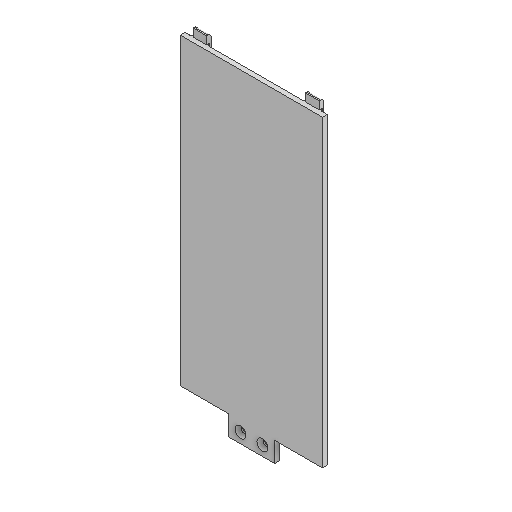
# Autodesk Inventor part: plate cover 2
Saved by Autodesk Inventor 2025.3 (Build 293356030, 356C)
## iProperties
Created: 2025-10-11
Part Number: plate cover 2
Material: 일반
Document SubType Name: Modeling
Designer: joseph
Density: 1 g/cm^3
Appearance: 기본값
Author: joseph
Autodesk Inventor part; units mm, degrees
ref_plane "YZ Plane" through (0, 0, 0) normal (1, 0, 0) x (0, 1, 0)
ref_plane "XZ Plane" through (0, 0, 0) normal (0, 1, 0) x (-1, 0, 0)
ref_plane "XY Plane" through (0, 0, 0) normal (0, 0, 1) x (1, 0, 0)
sketch "스케치1" plane through (0, 0, 0) normal (0, 0, 1) x (1, 0, 0)
  line L0 (0, 0) -> (90.5, 0)
  line L1 (90.5, 0) -> (90.5, 193.4)
  line L2 (90.5, 193.4) -> (0, 193.4)
  line L3 (0, 193.4) -> (0, 0)
  dimension "d0" = 90.5
  dimension "d1" = 193.4
  constraints: 8 end point, 2 parallel, 1 horizontal, 1 perpendicular
  measures "d0" distance of L2.end L1.end
  measures "d1" distance of L1.end L0.end
extrude "돌출1" add sketch "스케치1" along normal blind 3
sketch "스케치2" plane through (0, 0, 3) normal (0, 0, 1) x (1, 0, 0)
  line L0 (0, 0) -> (90.5, 0) projected
  line L1 (30.45, 0) -> (60.05, 0)
  line L2 (60.05, 0) -> (60.05, -12.8)
  line L3 (60.05, -12.8) -> (30.45, -12.8)
  line L4 (30.45, -12.8) -> (30.45, 0)
  circle A0 centre (38.25, -6.4) radius 1.5
  circle A1 centre (52.25, -6.4) radius 1.5
  point P0 (45.25, 0)
  dimension "d4" = 29.6
  dimension "d5" = 12.8
  dimension "d6" = 3
  dimension "d7" = 3
  dimension "d8" = 7.8
  dimension "d9" = 7.8
  constraints: 8 end point, 2 centre point, 2 midpoint, 2 parallel, 1 horizontal, 1 perpendicular, 1 point on line
  measures "d4" distance of L2.end L3.end
  measures "d5" distance of L1.end L2.end
  measures "d6" diameter of A0
  measures "d7" diameter of A1
  measures "d8" horizontal distance of L3.end A0.centre
  measures "d9" distance from line of L2 A1.centre
extrude "돌출2" add sketch "스케치2" against normal blind 3
sketch "스케치3" plane through (0, 193.4, 0) normal (0, 1, 0) x (1, 0, 0)
  line L0 (90.5, 0) -> (0, 0) projected
  line L1 (0, 0) -> (0, -3) projected
  line L2 (90.5, -3) -> (0, -3) projected
  line L3 (90.5, 0) -> (90.5, -3) projected
  line L4 (5.1, 0) -> (13.8, 0)
  line L5 (13.8, 0) -> (13.8, 2.8)
  line L6 (13.8, 2.8) -> (5.1, 2.8)
  line L7 (5.1, 2.8) -> (5.1, 0)
  line L8 (45.25, -3) -> (45.25, 0) construction
  line L9 (0, 0) -> (90.5, 0)
  line L10 (0, -3) -> (90.5, -3)
  line L11 (85.4, 0) -> (76.7, 0)
  line L12 (76.7, 0) -> (76.7, 2.8)
  line L13 (76.7, 2.8) -> (85.4, 2.8)
  line L14 (85.4, 2.8) -> (85.4, 0)
  dimension "d12" = 8.7
  dimension "d13" = 2.8
  dimension "d14" = 5.1
  constraints: 22 end point, 8 symmetric about line, 2 midpoint, 2 parallel, 2 point on line, 1 horizontal, 1 perpendicular
  measures "d12" distance of L6.end L5.end
  measures "d13" distance of L5.end L4.end
  measures "d14" horizontal distance of point (0, 0) L6.end
extrude "돌출3" add sketch "스케치3" against normal blind 20 contours L0 L12 L13 L14 | L0 L7 L6 L5
sketch "스케치4" plane through (0, 193.4, 3) normal (0, 1, 0) x (1, 0, 0)
  line L0 (5.1, 3) -> (5.1, 5.8) projected
  line L1 (13.8, 5.8) -> (13.8, 3) projected
  line L2 (5.1, 5.8) -> (13.8, 5.8)
  line L3 (13.8, 5.8) -> (13.8, 3)
  line L4 (13.8, 3) -> (5.1, 3)
  line L5 (5.1, 3) -> (5.1, 5.8)
  line L6 (85.4, 5.8) -> (76.7, 5.8) projected
  line L7 (76.7, 5.8) -> (85.4, 5.8)
  line L8 (85.4, 5.8) -> (85.4, 3)
  line L9 (85.4, 3) -> (76.7, 3)
  line L10 (76.7, 3) -> (76.7, 5.8)
  point P0 (0, 3)
  constraints: 16 end point, 4 parallel, 2 horizontal, 2 perpendicular, 1 point on line
extrude "돌출4" add sketch "스케치4" along normal blind 5
fillet "모깎기1" radius 2 8 edges at (9.45, 198.4, -2.8) (81.05, 198.4, -2.8) (5.1, 183.4, 0) (9.45, 173.4, 0) (13.8, 183.4, 0) (85.4, 183.4, 0) (81.05, 173.4, 0) (76.7, 183.4, 0)
fillet "모깎기2" radius 2 2 edges at (36.75, -6.4, 3) (50.75, -6.4, 3) inverted yes
